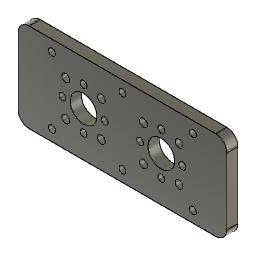
setupAssemblySingleJumpingLeg v1 (Autodesk Fusion 360 archive; units mm, degrees)
design "testBaseEncoder"
Autodesk Fusion 360 part; units mm, degrees
sketch "Sketch1" plane through (0, 0, 0) normal (0, 1, 0) x (1, 0, 0)
  circle A0 centre (101.4766, 0) radius 9.5 construction
  circle A1 centre (136.4766, 0) radius 9.5 construction
  circle A2 centre (101.4766, 0) radius 16.5 construction
  circle A3 centre (136.4766, 0) radius 16.5 construction
  circle A4 centre (101.4766, -9.5) radius 1.55
  circle A5 centre (110.9766, 0) radius 1.55
  circle A6 centre (101.4766, 9.5) radius 1.55
  circle A7 centre (91.9766, 0) radius 1.55
  circle A8 centre (136.4766, -9.5) radius 1.55
  circle A9 centre (145.9766, 0) radius 1.55
  circle A10 centre (136.4766, 9.5) radius 1.55
  circle A11 centre (126.9766, 0) radius 1.55
  circle A12 centre (118.9766, -15) radius 1.55
  circle A13 centre (118.9766, 15) radius 1.55
  line L0 (91.9766, -20) -> (145.9766, -20)
  line L1 (145.9766, 20) -> (91.9766, 20)
  line L2 (91.9766, 0) -> (145.9766, 0) construction
  circle A14 centre (101.4766, 0) radius 6
  circle A15 centre (136.4766, 0) radius 6
  line L3 (76.9766, 20) -> (160.9766, 20)
  line L4 (165.9766, 15) -> (165.9766, -15)
  line L5 (160.9766, -20) -> (76.9766, -20)
  line L6 (71.9766, -15) -> (71.9766, 15)
  line L7 (71.9766, 20) -> (165.9766, -20) construction
  line L8 (165.9766, 20) -> (71.9766, -20) construction
  arc A16 (71.9766, -15) -> (76.9766, -20) centre (76.9766, -15) ccw
  arc A17 (76.9766, 20) -> (71.9766, 15) centre (76.9766, 15) ccw
  arc A18 (165.9766, 15) -> (160.9766, 20) centre (160.9766, 15) ccw
  arc A19 (160.9766, -20) -> (165.9766, -15) centre (160.9766, -15) ccw
  line L9 (93.4766, -8) -> (109.4766, -8) construction
  line L10 (109.4766, -8) -> (109.4766, 8) construction
  line L11 (109.4766, 8) -> (93.4766, 8) construction
  line L12 (93.4766, 8) -> (93.4766, -8) construction
  line L13 (93.4766, -8) -> (109.4766, 8) construction
  line L14 (109.4766, -8) -> (93.4766, 8) construction
  line L15 (128.4766, -8) -> (144.4766, -8) construction
  line L16 (144.4766, -8) -> (144.4766, 8) construction
  line L17 (144.4766, 8) -> (128.4766, 8) construction
  line L18 (128.4766, 8) -> (128.4766, -8) construction
  line L19 (128.4766, -8) -> (144.4766, 8) construction
  line L20 (144.4766, -8) -> (128.4766, 8) construction
  circle A20 centre (93.4766, -8) radius 1.75
  circle A21 centre (109.4766, -8) radius 1.75
  circle A22 centre (93.4766, 8) radius 1.75
  circle A23 centre (109.4766, 8) radius 1.75
  circle A24 centre (128.4766, -8) radius 1.75
  circle A25 centre (144.4766, -8) radius 1.75
  circle A26 centre (128.4766, 8) radius 1.75
  circle A27 centre (144.4766, 8) radius 1.75
  circle A28 centre (87.2266, -15) radius 1.55
  circle A29 centre (87.2266, 15) radius 1.55
  circle A30 centre (150.7266, -15) radius 1.55
  circle A31 centre (150.7266, 15) radius 1.55
  point P0 (101.4766, 0)
  point P1 (136.4766, 0)
  point P2 (118.9766, 0)
  point P3 (101.4766, 0)
  point P4 (136.4766, 0)
  point P5 (118.9766, 0)
  point P6 (101.4766, 0)
  point P7 (136.4766, 0)
  dimension "d1" = 19
  dimension "d3" = 33
  dimension "d4" = 33
  dimension "d6" = 35
  dimension "d7" = 3.1
  dimension "d9" = 360
  dimension "d10" = 3.1
  dimension "d12" = 360
  dimension "d17" = 17.5
  dimension "d18" = 3.1
  dimension "d19" = 3.1
  dimension "d24" = 12
  dimension "d25" = 12
  dimension "d38" = 94
  dimension "d39" = 40
  dimension "d40" = 5
  dimension "d45" = 16
  dimension "d46" = 16
  dimension "d47" = 16
  dimension "d48" = 16
  dimension "d49" = 3.5
  dimension "d50" = 3.5
  dimension "d51" = 3.5
  dimension "d52" = 3.5
  dimension "d53" = 3.5
  dimension "d54" = 3.5
  dimension "d55" = 3.5
  dimension "d56" = 3.5
  dimension "d57" = 3.1
  dimension "d58" = 3.1
  dimension "d59" = 3.1
  dimension "d60" = 3.1
  dimension "d61" = 15
  dimension "d62" = 15
  dimension "d63" = 15
  dimension "d64" = 15
  dimension "d65" = 31.75
  dimension "d66" = 31.75
  dimension "d67" = 31.75
  dimension "d68" = 31.75
  constraint horizontal P6 P7
  constraint coincident P6 P0
  constraint coincident P7 P1
  constraint coincident P6 P3
  constraint coincident P7 P4
  constraint coincident A0 A4.centre
  constraint coincident A1 A8.centre
  constraint parallel L0 L1
  constraint coincident A9.centre L2.end
  constraint horizontal L2
  constraint coincident A7.centre L2.start
  constraint concentric A2 A14
  constraint concentric A3 A15
  constraint horizontal L3
  constraint perpendicular L3 L4
  constraint parallel L3 L5
  constraint parallel L4 L6
  constraint coincident L7 P5
  constraint coincident L8 P5
  constraint coincident P5 P2
  constraint coincident L8.end L6
  constraint coincident L8.end L5
  constraint tangent L6 A16
  constraint tangent L5 A16
  constraint coincident L7.start L6
  constraint coincident L7.start L3
  constraint tangent L6 A17
  constraint tangent L3 A17
  constraint equal A16 A17
  constraint coincident L8.start L3
  constraint coincident L8.start L4
  constraint tangent L3 A18
  constraint tangent L4 A18
  constraint equal A16 A18
  constraint coincident L7.end L4
  constraint coincident L7.end L5
  constraint tangent L4 A19
  constraint tangent L5 A19
  constraint equal A16 A19
  constraint horizontal L9
  constraint perpendicular L9 L10
  constraint parallel L9 L11
  constraint parallel L10 L12
  constraint coincident L13 P6
  constraint coincident L14 P6
  constraint horizontal L15
  constraint perpendicular L15 L16
  constraint parallel L15 L17
  constraint parallel L16 L18
  constraint coincident L19 P7
  constraint coincident L20 P7
  constraint coincident L9.start L12.end
  constraint coincident L9.end L10.start
  constraint coincident L11.end L12.start
  constraint coincident L10.end L11.start
  constraint coincident L15.start L18.end
  constraint coincident L15.end L16.start
  constraint coincident L17.end L18.start
  constraint coincident L16.end L17.start
  measures "d1" diameter of A0
  measures "d3" diameter of A2
  measures "d4" diameter of A3
  measures "d6" distance of P0 P7
  measures "d7" diameter of A4
  measures "d10" diameter of A8
  measures "d17" distance of P6 P5
  measures "d18" diameter of A12
  measures "d19" diameter of A13
  measures "d24" diameter of A14
  measures "d25" diameter of A15
  measures "d38" distance of L7.end L8.end
  measures "d39" distance of L8.start L7.end
  measures "d40" radius of A16
  measures "d45" distance of L10.end L11.end
  measures "d46" distance of L9.end L10.end
  measures "d47" distance of L16.end L17.end
  measures "d48" distance of L15.end L16.end
  measures "d49" diameter of A20
  measures "d50" diameter of A21
  measures "d51" diameter of A22
  measures "d52" diameter of A23
  measures "d53" diameter of A24
  measures "d54" diameter of A25
  measures "d55" diameter of A26
  measures "d56" diameter of A27
  measures "d57" diameter of A28
  measures "d58" diameter of A29
  measures "d59" diameter of A30
  measures "d60" diameter of A31
  measures "d61" vertical distance of P5 A28.centre
  measures "d62" vertical distance of P5 A29.centre
  measures "d63" vertical distance of P5 A30.centre
  measures "d64" vertical distance of P5 A31.centre
  measures "d65" horizontal distance of P5 A28.centre
  measures "d66" horizontal distance of P5 A30.centre
  measures "d67" horizontal distance of P5 A31.centre
  measures "d68" horizontal distance of P5 A29.centre
extrude "Extrude1" add sketch "Sketch1" along normal blind 5
equation "d17 = d6 / 2"
equation "d49 = d54"
equation "d50 = d54"
equation "d51 = d54"
equation "d52 = d54"
equation "d53 = d54"
equation "d55 = d54"
equation "d56 = d54"
equation "d61 = d63"
equation "d62 = d63"
equation "d64 = d63"
equation "d66 = d65"
equation "d67 = d65"
equation "d68 = d65"

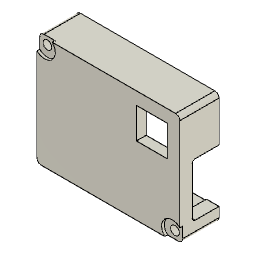
design "Top_PCB_Cover"
Autodesk Fusion 360 part; units mm, degrees
sketch "Sketch1" plane through (0, 0, 0) normal (0, 1, 0) x (1, 0, 0)
  line L0 (0, 0) -> (41, 0) construction
  line L1 (41, 0) -> (41, -30) construction
  line L2 (41, -30) -> (0, -30) construction
  line L3 (0, -30) -> (0, 0) construction
  line L4 (-0.5, 0.5) -> (41.5, 0.5)
  line L5 (41.5, 0.5) -> (41.5, -30.5)
  line L6 (41.5, -30.5) -> (-0.5, -30.5)
  line L7 (-0.5, -30.5) -> (-0.5, 0.5)
  line L8 (-5, 5) -> (46, 5)
  line L9 (46, 5) -> (46, -35)
  line L10 (46, -35) -> (-5, -35)
  line L11 (-5, -35) -> (-5, 5)
  line L12 (30.5, -30.5) -> (30.5, -19.5)
  line L13 (30.5, -19.5) -> (41.5, -19.5)
  circle A0 centre (43.3031, 2.3031) radius 1.55
  circle A1 centre (-2.3031, -32.3031) radius 1.55
  circle A2 centre (-2.3031, -32.3031) radius 3.814
  circle A3 centre (43.3031, 2.3031) radius 3.814
  dimension "d1" = 41
  dimension "d2" = 30
  dimension "d3" = -0.5
  dimension "d4" = -5
  dimension "d5" = 11
  dimension "d6" = 11
  dimension "d7" = 3.1
  dimension "d8" = 3.1
  dimension "d22" = 2.55
  dimension "d23" = 2.55
  dimension "d30" = 7.6279
  dimension "d32" = 3.814
  dimension "d33" = 7.6279
  constraint horizontal L0
  constraint vertical L1
  constraint horizontal L2
  constraint vertical L3
  constraint coincident L0.start L3.end
  constraint coincident L6 L12.start
  constraint perpendicular L2 L12
  constraint coincident L5 L13.end
  constraint perpendicular L5 L13
  constraint concentric A1 A2
  constraint concentric A0 A3
  measures "d1" distance of L0.start L0.end
  measures "d2" distance of L0.start L2.end
  measures "d5" distance of L5 L12
  measures "d6" distance of L6 L13
  measures "d7" diameter of A0
  measures "d8" diameter of A1
  measures "d22" distance of L4.end A0.centre
  measures "d23" distance of L6.end A1.centre
  measures "d30" diameter of A2
  measures "d32" distance of L8.end A0.centre
  measures "d33" diameter of A3
extrude "Extrude1" add sketch "Sketch1" along normal blind 3.5 contours L4 L5 L6 L7 L12 L13 A2 A3 | L4 L5 A3 | L6 L7 A2
extrude "Extrude2" add sketch "Sketch1" along normal blind 14 contours L4 L7 L8 L11 A2 A3 | L4 L5 L8 L9 A3 | L6 L7 L10 L11 A2 | L5 L6 L9 L10 A2 A3
fillet "Fillet1" radius 1.5 4 edges at (46, 7, -5) (46, 7, 35) (-5, 7, -5) (-5, 7, 35)
ref_plane "WorkPlane1" through (20.5, 14, 15) normal (0, 1, 0) x (1, 0, 0)
sketch "Sketch2" plane through (0, 14, 0) normal (0, 1, 0) x (1, 0, 0)
  line L0 (41, -30) -> (0, -30)
  line L1 (41, 0) -> (41, -30)
  line L2 (41.5, 0.5) -> (41.5, -30.5)
  line L3 (41.5, -30.5) -> (-0.5, -30.5)
  line L4 (0, -30) -> (0, 0)
  line L5 (-0.5, -30.5) -> (-0.5, 0.5)
  line L6 (0, 0) -> (41, 0)
  line L7 (-0.5, 0.5) -> (41.5, 0.5)
  line L8 (-5, 5) -> (46, 5)
  line L9 (46, 5) -> (46, -35)
  line L10 (-5, -35) -> (-5, 5)
  line L11 (46, -35) -> (-5, -35)
  circle A0 centre (43.3031, 2.3031) radius 1.55
  circle A1 centre (-2.3031, -32.3031) radius 1.55
  line L12 (46, 0) -> (41.5, 0)
  line L13 (41.5, 0) -> (41.5, -19)
  line L14 (41.5, -19) -> (46, -19)
  line L15 (46, -19) -> (46, 0)
  line L16 (-0.5, 0) -> (-5, 0)
  line L17 (-5, 0) -> (-5, -19)
  line L18 (-5, -19) -> (-0.5, -19)
  line L19 (-0.5, -19) -> (-0.5, 0)
  line L20 (-5, 5) -> (13, 5)
  line L21 (13, 5) -> (13, 0)
  line L22 (13, 0) -> (-5, 0)
  line L23 (-5, 0) -> (-5, 5)
  line L24 (-0.5, -30.5) -> (-5, -30.5)
  line L25 (-5, -30.5) -> (-5, -27.5)
  line L26 (-5, -27.5) -> (-0.5, -27.5)
  line L27 (-0.5, -27.5) -> (-0.5, -30.5)
  dimension "d16" = 19
  dimension "d17" = 19
  dimension "d18" = 18
  dimension "d19" = 5
  dimension "d28" = 34.6062
  dimension "d29" = 45.6062
  dimension "d36" = 3
  constraint horizontal L12
  constraint vertical L13
  constraint horizontal L14
  constraint vertical L15
  constraint coincident L9 L12.start
  constraint horizontal L16
  constraint vertical L17
  constraint horizontal L18
  constraint vertical L19
  constraint coincident L5 L16.start
  constraint horizontal L20
  constraint vertical L21
  constraint horizontal L22
  constraint vertical L23
  constraint coincident L8.start L10.end
  constraint horizontal L24
  constraint vertical L25
  constraint horizontal L26
  constraint vertical L27
  constraint coincident L3.end L5.start
  measures "d16" distance of L12.start L14.end
  measures "d17" distance of L16.start L18.end
  measures "d18" distance of L8.start L20.end
  measures "d19" distance of L8.start L16.end
  measures "d28" vertical distance of A0.centre A1.centre
  measures "d29" horizontal distance of A0.centre A1.centre
  measures "d36" distance of L3.end L26.end
extrude "Extrude3" cut sketch "Sketch2" against normal blind 9.5 contours L5 L7 L8 L10 L16 L20 L21 L22 L23 | L5 L10 L16 L17 L18 L19 L22 | L5 L10 L18 L26 | L2 L9 L12 L13 L14 L15
extrude "Extrude4" cut sketch "Sketch1" along normal blind 1 contours L4 L5 L8 L9 A3 | L4 L5 A3 | L6 L7 A2 | L6 L7 L10 L11 A2 | L8 A3 | L11 A2 | L9 A3 | L10 A2
fillet "Fillet3" radius 1 4 edges at (-2.75, 4.5, 27.5) (13, 4.5, -2.75) (43.75, 4.5, 19) (43.75, 4.5, 0)
equation "d6 = d5"
equation "d9 = TOTAL_HEIGHT - WIRE_HEIGHT - 1 mm"
equation "d11 = TOTAL_HEIGHT"
equation "d20 = -WIRE_HEIGHT"
equation "d22 = d7 / 2 + 1 mm"
equation "d23 = d8 / 2 + 1 mm"
equation "TOTAL_HEIGHT = 14 mm"
equation "WIRE_HEIGHT = 9.5 mm"
equation "d30 = d33"
equation "d33 = d32 * 2"

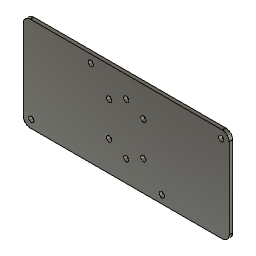
design "STMBackPlateNew"
Autodesk Fusion 360 part; units mm, degrees
sketch "Sketch1" plane through (0, 0, 0) normal (0, 1, 0) x (1, 0, 0)
  line L0 (0, 0) -> (120, 0)
  line L1 (120, 0) -> (120, -55)
  line L2 (120, -55) -> (0, -55)
  line L3 (0, -55) -> (0, 0)
  line L4 (50, -37.5) -> (70, -37.5) construction
  line L5 (70, -37.5) -> (70, -17.5) construction
  line L6 (70, -17.5) -> (50, -17.5) construction
  line L7 (50, -17.5) -> (50, -37.5) construction
  line L8 (50, -37.5) -> (70, -17.5) construction
  line L9 (70, -37.5) -> (50, -17.5) construction
  line L10 (4.697, -50.303) -> (39.303, -50.303) construction
  line L11 (39.303, -50.303) -> (39.303, -4.697) construction
  line L12 (39.303, -4.697) -> (4.697, -4.697) construction
  line L13 (4.697, -4.697) -> (4.697, -50.303) construction
  line L14 (4.697, -50.303) -> (39.303, -4.697) construction
  line L15 (39.303, -50.303) -> (4.697, -4.697) construction
  circle A0 centre (39.303, -50.303) radius 1.55
  circle A1 centre (4.697, -4.697) radius 1.55
  circle A2 centre (50, -37.5) radius 1.55
  circle A3 centre (70, -37.5) radius 1.55
  circle A4 centre (50, -17.5) radius 1.55
  line L16 (60, -27.5) -> (60, -45)
  line L17 (115.303, -50.303) -> (80.697, -50.303)
  line L18 (80.697, -50.303) -> (80.697, -4.697)
  line L19 (80.697, -4.697) -> (115.303, -4.697)
  line L20 (115.303, -4.697) -> (115.303, -50.303)
  line L21 (115.303, -50.303) -> (80.697, -4.697) construction
  line L22 (80.697, -50.303) -> (115.303, -4.697) construction
  circle A5 centre (115.303, -50.303) radius 1.55
  circle A6 centre (80.697, -4.697) radius 1.55
  circle A7 centre (60, -42.5) radius 1.55
  circle A8 centre (60, -12.5) radius 1.55
  circle A9 centre (70, -17.5) radius 1.55
  line L23 (0.697, -54.303) -> (43.303, -54.303) construction
  line L24 (43.303, -54.303) -> (43.303, -0.697) construction
  line L25 (43.303, -0.697) -> (0.697, -0.697) construction
  line L26 (0.697, -0.697) -> (0.697, -54.303) construction
  line L27 (76.697, -0.697) -> (119.303, -0.697) construction
  line L28 (119.303, -0.697) -> (119.303, -54.303) construction
  line L29 (119.303, -54.303) -> (76.697, -54.303) construction
  line L30 (76.697, -54.303) -> (76.697, -0.697) construction
  circle A10 centre (50, -37.5) radius 3.5 construction
  circle A11 centre (70, -37.5) radius 3.5 construction
  circle A12 centre (50, -17.5) radius 3.5 construction
  circle A13 centre (70, -17.5) radius 3.5 construction
  point P0 (60, -27.5)
  point P1 (60, -27.5)
  point P2 (22, -27.5)
  point P3 (98, -27.5)
  dimension "d1" = 120
  dimension "d2" = 55
  dimension "d3" = 20
  dimension "d4" = 20
  dimension "d5" = 34.606
  dimension "d6" = 45.606
  dimension "d7" = 22
  dimension "d8" = 27.5
  dimension "d9" = 60
  dimension "d10" = 3.1
  dimension "d11" = 3.1
  dimension "d12" = 27.5
  dimension "d13" = 3.1
  dimension "d14" = 3.1
  dimension "d15" = 3.1
  dimension "d16" = 34.606
  dimension "d17" = 45.606
  dimension "d18" = 22
  dimension "d19" = 27.5
  dimension "d20" = 3.1
  dimension "d21" = 3.1
  dimension "d22" = 3.1
  dimension "d23" = 3.1
  dimension "d24" = 15
  dimension "d25" = 15
  dimension "d26" = 3.1
  dimension "d31" = 4
  dimension "d32" = -4
  dimension "d33" = 7
  dimension "d34" = 7
  dimension "d35" = 7
  dimension "d36" = 7
  constraint horizontal L0
  constraint vertical L1
  constraint horizontal L2
  constraint vertical L3
  constraint coincident L0.start L3.end
  constraint horizontal L4
  constraint perpendicular L4 L5
  constraint parallel L4 L6
  constraint parallel L5 L7
  constraint coincident L8 P1
  constraint coincident L9 P1
  constraint coincident P1 P0
  constraint horizontal L10
  constraint perpendicular L10 L11
  constraint parallel L10 L12
  constraint parallel L11 L13
  constraint coincident L14 P2
  constraint coincident L15 P2
  constraint coincident L10.end L11.start
  constraint coincident L12.end L13.start
  constraint coincident L4.start L7.end
  constraint coincident L4.end L5.start
  constraint coincident L6.end L7.start
  constraint parallel L5 L16
  constraint horizontal L17
  constraint perpendicular L17 L18
  constraint parallel L17 L19
  constraint parallel L18 L20
  constraint coincident L21 P3
  constraint coincident L22 P3
  constraint coincident L17.start L20.end
  constraint coincident L18.end L19.start
  constraint coincident L16 A7.centre
  constraint coincident L5.end L6.start
  constraint concentric A2 A10
  constraint concentric A3 A11
  constraint concentric A4 A12
  constraint concentric A9 A13
  measures "d1" distance of L0.start L0.end
  measures "d2" distance of L0.start L2.end
  measures "d3" distance of L5.end L6.end
  measures "d4" distance of L4.end L5.end
  measures "d5" distance of L11.end L12.end
  measures "d6" distance of L10.end L11.end
  measures "d7" distance of L3 P2
  measures "d8" distance of L0 P1
  measures "d9" distance of L3 P1
  measures "d10" diameter of A0
  measures "d11" diameter of A1
  measures "d12" distance of L0 P2
  measures "d13" diameter of A2 L18.end
  measures "d14" diameter of A3 L18.end
  measures "d15" diameter of A4 L18.end
  measures "d16" distance of L18.end L19.end
  measures "d17" distance of L17.end L18.end
  measures "d18" distance of L1 P3
  measures "d19" distance of L0 P3
  measures "d20" diameter of A5
  measures "d21" diameter of A6
  measures "d22" diameter of A7
  measures "d23" diameter of A8
  measures "d24" distance of P1 A7.centre
  measures "d25" distance of P1 A8.centre
  measures "d26" diameter of A9 L18.end
  measures "d33" diameter of A10 L18.end
  measures "d34" diameter of A11 L18.end
  measures "d35" diameter of A12 L18.end
  measures "d36" diameter of A13 L18.end
extrude "Extrude1" add sketch "Sketch1" along normal blind 2 contours L0 L1 L2 L3 | L17 L18 L19 L20 A5 A6
fillet "Fillet1" radius 4 4 edges at (120, 1, 55) (120, 1, 0) (0, 1, 55) (0, 1, 0)
equation "d8 = d2 / 2"
equation "d9 = d1 / 2"
equation "d12 = d2 / 2"
equation "d18 = d7"
equation "d19 = d12"
equation "d25 = d24"
